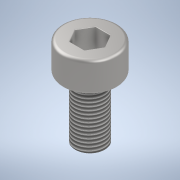
# Autodesk Inventor part: L Bolt M3 x 6 Stainless Steel
Saved by Autodesk Inventor 2020 (Build 240168000, 168)
## iProperties
Created: 2023-01-23
Part Number: L Bolt M3 x 6 Stainless Steel
Material: Generic
Document SubType Name: Modeling
Designer: Thompson Ray
Density: 1 g/cm^3
Appearance: Stainless - Brushed
Author: Thompson Ray
Autodesk Inventor part; units mm, degrees
ref_plane "YZ Plane" through (0, 0, 0) normal (1, 0, 0) x (0, 1, 0)
ref_plane "XZ Plane" through (0, 0, 0) normal (0, 1, 0) x (-1, 0, 0)
ref_plane "XY Plane" through (0, 0, 0) normal (0, 0, 1) x (1, 0, 0)
sketch "Sketch1" plane through (0, 0, 0) normal (0, 1, 0) x (-1, 0, 0)
  circle A0 centre (0, 0) radius 1.5
  dimension "d1" = 3
  constraints: 1 centre point, 1 coincident
  measures "d1" diameter of A0
extrude "Extrusion1" add sketch "Sketch1" along normal blind 6
sketch "Sketch2" plane through (0, 6, 0) normal (0, 1, 0) x (1, 0, 0)
  circle A0 centre (0, 0) radius 2.75
  dimension "d4" = 5.5
  constraints: 1 centre point, 1 coincident
  measures "d4" diameter of A0
extrude "Extrusion2" add sketch "Sketch2" along normal blind 3
sketch "Sketch3" plane through (0, 9, 0) normal (0, 1, 0) x (1, 0, 0)
  line L0 (1.5, 0) -> (0.75, -1.299)
  line L1 (0.75, -1.299) -> (-0.75, -1.299)
  line L2 (-0.75, -1.299) -> (-1.5, 0)
  line L3 (-1.5, 0) -> (-0.75, 1.299)
  line L4 (-0.75, 1.299) -> (0.75, 1.299)
  line L5 (0.75, 1.299) -> (1.5, 0)
  point P0 (0, 0)
  point P1 (0, 0)
  dimension "d7" = 1.5
  constraints: 12 end point, 1 coincident, 13 other
  measures "d7" distance of point (0, 0) L0.start
extrude "Extrusion3" cut sketch "Sketch3" against normal blind 2
thread "Thread1" size "M3x0.35" class "6g" standard "ISO Metric profile" length 6
fillet "Fillet1" radius 0.3 2 edges at (-2.75, 6, 0) (-2.75, 9, 0)
chamfer "Chamfer1" distance 0.05 angle 45 1 edges at (1.5, 0, 0)
chamfer "Chamfer2" distance 0.05 angle 45 1 edges at (1.5, 6, 0)
fillet "Fillet2" radius 0.05 12 edges at (0, 9, -1.299) (1.125, 9, -0.6495) (1.125, 9, 0.6495) (0, 9, 1.299) (-1.125, 9, 0.6495) (-1.125, 9, -0.6495) (0, 7, -1.299) (1.125, 7, -0.6495) (1.125, 7, 0.6495) (-1.125, 7, -0.6495) (-1.125, 7, 0.6495) (0, 7, 1.299)
sketch "Sketch4" plane through (0, 0, 0) normal (0, -1, 0) x (1, 0, 0)
  circle A0 centre (0, 0) radius 1.425
  dimension "d21" = 2.85
  constraints: 1 centre point, 1 coincident
  measures "d21" diameter of A0
extrude "Extrusion4" cut sketch "Sketch4" against normal blind 0.1
chamfer "Chamfer3" distance 0.05 angle 45 1 edges at (-1.425, 0.1, 0)
body "Solid1"
